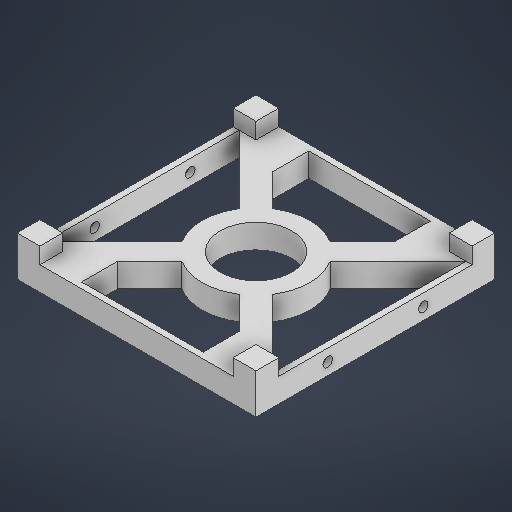
# Autodesk Inventor part: Top&Bottom
Saved by Autodesk Inventor 2026.1 (Build 301233020, 233B)
## iProperties
Created: 2025-10-16
Part Number: Top&Bottom
Material: Generic
Document SubType Name: Modeling
Designer: scott
Density: 1 g/cm^3
Appearance: Default
Author: scott
Autodesk Inventor part; units mm, degrees
ref_plane "YZ Plane" through (0, 0, 0) normal (1, 0, 0) x (0, 1, 0)
ref_plane "XZ Plane" through (0, 0, 0) normal (0, 1, 0) x (-1, 0, 0)
ref_plane "XY Plane" through (0, 0, 0) normal (0, 0, 1) x (1, 0, 0)
sketch "Sketch1" plane through (0, 0, 0) normal (0, 1, 0) x (-1, 0, 0)
  line L0 (50, 50) -> (-50, 50)
  line L1 (-50, 50) -> (-50, -50)
  line L2 (-50, -50) -> (50, -50)
  line L3 (50, -50) -> (50, 50)
  line L4 (-50, 50) -> (50, -50) construction
  line L5 (-47.5, 47.5) -> (47.5, 47.5)
  line L6 (47.5, 47.5) -> (47.5, -47.5)
  line L7 (47.5, -47.5) -> (-47.5, -47.5)
  line L8 (-47.5, -47.5) -> (-47.5, 47.5)
  line L9 (-47.5, 47.5) -> (47.5, -47.5) construction
  circle A0 centre (0, 0) radius 22.5
  circle A1 centre (0, 0) radius 15
  line L10 (40.4289, 47.5) -> (11.9766, 19.0476)
  line L11 (47.5, 40.4289) -> (19.0476, 11.9765)
  line L12 (-47.5, 40.4289) -> (-19.0476, 11.9766)
  line L13 (-40.4289, 47.5) -> (-11.9765, 19.0476)
  line L14 (-40.4289, -47.5) -> (-11.9766, -19.0476)
  line L15 (-47.5, -40.4289) -> (-19.0476, -11.9765)
  line L16 (47.5, -40.4289) -> (19.0476, -11.9766)
  line L17 (40.4289, -47.5) -> (11.9765, -19.0476)
  circle A2 centre (35, -35) radius 2
  circle A3 centre (35, 35) radius 2
  circle A4 centre (-35, 35) radius 2
  circle A5 centre (-35, -35) radius 2
  point P0 (19.0476, -11.9766)
  point P1 (-11.9765, 19.0476)
  point P2 (-11.9766, -19.0476)
  point P3 (11.9765, -19.0476)
  dimension "d0" = 100
  dimension "d1" = 100
  dimension "d2" = 95
  dimension "d3" = 95
  dimension "d9" = 30
  dimension "d10" = 7.5
  dimension "d11" = 10
  dimension "d12" = 7.0711
  dimension "d13" = 7.0711
  dimension "d16" = 360
  dimension "d23" = 4
  dimension "d24" = 35
  dimension "d27" = 360
  constraints: 36 end point, 6 centre point, 4 parallel, 3 point on line, 2 horizontal, 2 midpoint, 2 perpendicular, 2 point on circle, 1 coincident, 34 other
  measures "d0" distance of L2.end L1.end
  measures "d1" distance of L1.end L0.end
  measures "d2" distance of L6.end L7.end
  measures "d3" distance of L5.end L6.end
  measures "d9" diameter of A1
  measures "d10" radial gap between concentric circles of A0 A1
  measures "d11" distance between parallel lines of L11 L10
  measures "d12" distance of L5.end L10.start
  measures "d13" distance of L11.start L5.end
  measures "d23" diameter of A2
  measures "d24" horizontal distance of A2.centre A1.centre
extrude "Extrusion1" add sketch "Sketch1" along normal blind 10 contours L3 L2 L1 L0 | L5 L13 A0 L12 L8 | L5 L6 L11 A0 L10 | A0 | L15 A0 L14 L7 L8 | L6 L7 L17 A0 L16 | A2 | A3 | A4 | A5
sketch "Sketch3" plane through (0, 10, 0) normal (0, 1, 0) x (1, 0, 0)
  line L0 (-50, -50) -> (-40.43, -50)
  line L1 (-40.43, -50) -> (-40.43, -40.43)
  line L2 (-40.43, -40.43) -> (-50, -40.43)
  line L3 (-50, -40.43) -> (-50, -50)
  line L4 (40.43, -40.43) -> (40.43, -50)
  line L5 (40.43, -50) -> (50, -50)
  line L6 (50, -40.43) -> (40.43, -40.43)
  line L7 (50, -50) -> (50, -40.43)
  line L8 (40.43, 40.43) -> (50, 40.43)
  line L9 (50, 40.43) -> (50, 50)
  line L10 (40.43, 50) -> (40.43, 40.43)
  line L11 (50, 50) -> (40.43, 50)
  line L12 (-40.43, 40.43) -> (-40.43, 50)
  line L13 (-40.43, 50) -> (-50, 50)
  line L14 (-50, 40.43) -> (-40.43, 40.43)
  line L15 (-50, 50) -> (-50, 40.43)
  point P0 (0, 0)
  dimension "d29" = 9.57
  dimension "d30" = 9.57
  dimension "d33" = 360
  constraints: 32 end point, 2 parallel, 1 horizontal, 1 perpendicular, 33 other
  measures "d29" distance of L2.end L1.end
  measures "d30" distance of L1.end L0.end
extrude "Extrusion2" add sketch "Sketch3" along normal blind 6.75
sketch "Sketch4" plane through (-50, 0, -50) normal (-1, 0, 0) x (0, 0, 1)
  circle A0 centre (30, 5) radius 2
  line L0 (0, 0) -> (0, 16.75) projected
  circle A1 centre (70, 5) radius 2
  line L1 (100, 0) -> (100, 16.75) projected
  point P0 (50, 0)
  dimension "d37" = 4
  dimension "d38" = 30
  dimension "d39" = 4
  dimension "d40" = 30
  constraints: 2 centre point
  measures "d37" diameter of A0
  measures "d38" distance from line of A0.centre L0
  measures "d39" diameter of A1
  measures "d40" distance from line of A1.centre L1
extrude "Extrusion3" cut sketch "Sketch4" against normal blind 6.75
sketch "Sketch5" plane through (50, 0, 50) normal (1, 0, 0) x (0, 0, -1)
  circle A0 centre (30, 5) radius 2
  line L0 (0, 0) -> (0, 16.75) projected
  circle A1 centre (70, 5) radius 2
  line L1 (100, 0) -> (100, 16.75) projected
  point P0 (50, 0)
  dimension "d43" = 4
  dimension "d44" = 30
  dimension "d45" = 4
  dimension "d46" = 30
  constraints: 2 centre point
  measures "d43" diameter of A0
  measures "d44" distance from line of A0.centre L0
  measures "d45" diameter of A1
  measures "d46" distance from line of A1.centre L1
extrude "Extrusion4" cut sketch "Sketch5" against normal blind 6.75
sketch "Sketch6" plane through (0, 0, 0) normal (0, -1, 0) x (1, 0, 0)
  line L0 (35, 45) -> (-35, 45)
  line L1 (-35, 45) -> (-35, -45)
  line L2 (-35, -45) -> (35, -45)
  line L3 (35, -45) -> (35, 45)
  line L4 (35, 45) -> (-35, -45) construction
  line L5 (-35, 45) -> (35, -45) construction
  line L6 (40.4289, 47.5) -> (25.4289, 47.5)
  line L7 (40.4289, 47.5) -> (-40.4289, 47.5) projected
  line L8 (25.4289, 47.5) -> (25.4289, 32.5)
  line L9 (25.4289, 32.5) -> (40.4289, 47.5)
  line L10 (40.4289, -47.5) -> (11.9766, -19.0476) projected
  line L11 (40.4289, -47.5) -> (25.4289, -47.5)
  line L12 (-40.4289, -47.5) -> (40.4289, -47.5) projected
  line L13 (-40.4289, 47.5) -> (-25.4289, 47.5)
  line L14 (-40.4289, -47.5) -> (-25.4289, -47.5)
  circle A0 centre (32.5, 42) radius 1.5
  circle A1 centre (32.5, -42) radius 1.5
  circle A2 centre (-33, -42) radius 1.5
  circle A3 centre (-33, 42) radius 1.5
  line L15 (-40.4289, -47.5) -> (-25.4289, -47.5)
  line L16 (-25.4289, -47.5) -> (-25.4289, -32.5)
  line L17 (-25.4289, -32.5) -> (-40.4289, -47.5)
  line L18 (-40.4289, 47.5) -> (-25.4289, 47.5)
  line L19 (-40.4289, 47.5) -> (-25.4289, 47.5)
  line L20 (-40.4289, 47.5) -> (-25.4289, 47.5) construction
  line L21 (-25.4289, 47.5) -> (-25.4289, 32.5)
  line L22 (-25.4289, 32.5) -> (-40.4289, 47.5)
  line L23 (25.4289, -47.5) -> (25.4289, -32.5)
  line L24 (25.4289, -47.5) -> (40.4289, -47.5) construction
  line L25 (25.4289, -32.5) -> (40.4289, -47.5)
  point P0 (0, 0)
  point P1 (-34.4058, -41.4769)
  point P2 (-33.5231, -40.5942)
  point P3 (-33.5231, 40.5942)
  point P4 (-34.4058, 41.4769)
  dimension "d49" = 70
  dimension "d50" = 90
  dimension "d51" = 15
  dimension "d52" = 15
  dimension "d53" = 90
  dimension "d54" = 15
  dimension "d56" = 15
  dimension "d58" = 15
  dimension "d59" = 3
  dimension "d60" = 2.5
  dimension "d61" = 3
  dimension "d62" = 3
  dimension "d63" = 3
  dimension "d64" = 2.5
  dimension "d65" = 3
  dimension "d66" = 3
  dimension "d67" = 2
  dimension "d68" = 3
  dimension "d69" = 3
  dimension "d70" = 2
  dimension "d71" = 15
  dimension "d72" = 15
  dimension "d73" = 0
  dimension "d74" = 15
  dimension "d75" = 90
  dimension "d76" = 15
  dimension "d77" = 90
  constraints: 46 end point, 4 centre point, 4 horizontal, 4 perpendicular, 4 point on line, 2 collinear, 2 equal length, 2 midpoint, 2 parallel, 1 vertical
  measures "d49" distance of L2.end L1.end
  measures "d50" distance of L1.end L0.end
  measures "d51" distance of L6.start L6.end
  measures "d52" distance of L6.end L8.end
  measures "d53" angle of L8 L6
  measures "d54" distance of L10.start L11.end
  measures "d56" distance of L7.end L13.end
  measures "d58" distance of L12.start L14.end
  measures "d59" diameter of A0
  measures "d60" distance from line of L3 A0.centre
  measures "d61" distance from line of A0.centre L0
  measures "d62" diameter of A1
  measures "d63" distance from line of L2 A1.centre
  measures "d64" distance from line of L3 A1.centre
  measures "d65" diameter of A2
  measures "d66" distance from line of L2 A2.centre
  measures "d67" distance from line of A2.centre L1
  measures "d68" diameter of A3
  measures "d69" distance from line of L0 A3.centre
  measures "d70" distance from line of L1 A3.centre
  measures "d71" distance of L14.end L16.end
  measures "d72" distance of L7.end L13.end
  measures "d73" distance between parallel lines of L19 L20
  measures "d74" distance of L13.end L21.end
  measures "d75" angle of L19 L21
  measures "d76" distance of L11.end L23.end
  measures "d77" angle of L24 L23
extrude "Extrusion5" cut sketch "Sketch6" against normal blind 10 contours A3 L22 | A2 L17 picked at (-33.9131, 40.9363) picked at (-33.9131, -40.9363)
extrude "Extrusion6" add sketch "Sketch6" against normal blind 10 contours L3 L9 L8 L0 | L0 L8 L6 L9 L3 | L21 L22 A3 L1 L0 | L0 L1 L22 L7 L21 | L10 L11 L23 L2 L3 | L3 L2 L23 L10 | L17 A2 L16 L2 L1 | L1 L2 L16 L12 L17
sketch "Sketch8" plane through (0, 10, 0) normal (0, 1, 0) x (1, 0, 0)
  circle A0 centre (-33, 42) radius 1.5 projected
  circle A1 centre (-33, 42) radius 1.5
  circle A2 centre (32.5, 42) radius 1.5 projected
  circle A3 centre (32.5, 42) radius 1.5
  circle A4 centre (32.5, -42) radius 1.5 projected
  circle A5 centre (32.5, -42) radius 1.5
  circle A6 centre (-33, -42) radius 1.5
  point P0 (0, 0)
  constraints: 4 centre point, 3 coincident
extrude "Extrusion7" add sketch "Sketch8" against normal blind 4
equation "\"d18\" = d11"
body "Solid1"
